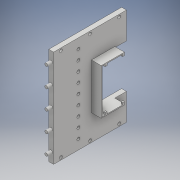
# Autodesk Inventor part: Front Plate V3
Saved by Autodesk Inventor 2017.3 (Build 213256000, 256)
## iProperties
Created: 2018-03-06
Part Number: Front Plate V3
Material: Generic
Document SubType Name: Modeling
Designer: Harsh Gupta
Density: 1 g/cm^3
Appearance: Default
Author: Harsh Gupta
Autodesk Inventor part; units mm, degrees
ref_plane "YZ Plane" through (0, 0, 0) normal (1, 0, 0) x (0, 1, 0)
sketch "Sketch2" plane through (0, 0, 0) normal (0, 1, 0) x (-1, 0, 0)
  line L0 (0, 0) -> (5, 0)
  line L1 (5, 0) -> (5, -100)
  line L2 (5, -100) -> (0, -100)
  line L3 (0, -100) -> (0, 0)
  dimension "d0" = 5
  dimension "d1" = 100
  constraints: 8 end point, 2 parallel, 1 horizontal, 1 perpendicular
  measures "d0" distance of L1.end L2.end
  measures "d1" distance of L0.end L1.end
extrude "Extrusion1" add sketch "Sketch2" along normal blind 75
sketch "Sketch4" plane through (0, 0, 0) normal (1, 0, 0) x (0, 0, -1)
  line L0 (0, 75) -> (100, 75) projected
  line L1 (27.5, 40) -> (72.5, 40)
  line L2 (72.5, 40) -> (72.5, 75)
  line L3 (72.5, 75) -> (27.5, 75)
  line L4 (27.5, 75) -> (27.5, 40)
  line L5 (100, 0) -> (100, 75) projected
  line L6 (0, 0) -> (100, 0) projected
  line L7 (0, 0) -> (0, 75) projected
  dimension "d9" = 27.5
  dimension "d11" = 40
  dimension "d12" = 45
  dimension "d13" = 27.5
  constraints: 8 end point, 2 parallel, 1 horizontal, 1 perpendicular, 1 point on line
  measures "d9" distance between parallel lines of L5 L2
  measures "d11" distance between parallel lines of L6 L1
  measures "d12" distance of L1.start L1.end
  measures "d13" distance between parallel lines of L7 L4
extrude "Extrusion3" cut sketch "Sketch4" against normal through all contours L0 L2 L1 L4
sketch "Sketch5" plane through (0, 0, 0) normal (1, 0, 0) x (0, 0, -1)
  line L0 (72.5, 43) -> (27.5, 43) projected
  line L1 (72.5, 63) -> (72.5, 43) projected
  line L2 (27.5, 63) -> (72.5, 63) projected
  line L3 (27.5, 43) -> (27.5, 63) projected
  circle A0 centre (28.5, 44) radius 0.75 projected
  circle A1 centre (28.5, 62) radius 0.75 projected
  circle A2 centre (71.5, 44) radius 0.75 projected
  circle A3 centre (71.5, 62) radius 0.75 projected
  line L4 (47.55, 45.5) -> (47.35, 45.5) projected
  line L5 (47.55, 45.5) -> (47.65, 45.6) projected
  line L6 (49.8, 45.6) -> (47.65, 45.6) projected
  line L7 (49.8, 45.6) -> (49.9, 45.5) projected
  line L8 (50.1, 45.5) -> (49.9, 45.5) projected
  line L9 (50.1, 45.5) -> (50.2, 45.6) projected
  line L10 (52.35, 45.6) -> (50.2, 45.6) projected
  line L11 (52.35, 45.6) -> (52.45, 45.5) projected
  line L12 (52.65, 45.5) -> (52.45, 45.5) projected
  line L13 (52.65, 45.5) -> (52.75, 45.6) projected
  line L14 (54.9, 45.6) -> (52.75, 45.6) projected
  line L15 (54.9, 45.6) -> (55, 45.5) projected
  line L16 (55, 43.2) -> (55, 45.5) projected
  line L17 (55, 43.2) -> (54.9, 43.1) projected
  line L18 (52.75, 43.1) -> (54.9, 43.1) projected
  line L19 (52.75, 43.1) -> (52.65, 43.2) projected
  line L20 (52.45, 43.2) -> (52.65, 43.2) projected
  line L21 (52.45, 43.2) -> (52.35, 43.1) projected
  line L22 (50.2, 43.1) -> (52.35, 43.1) projected
  line L23 (50.2, 43.1) -> (50.1, 43.2) projected
  line L24 (49.9, 43.2) -> (50.1, 43.2) projected
  line L25 (49.9, 43.2) -> (49.8, 43.1) projected
  line L26 (47.65, 43.1) -> (49.8, 43.1) projected
  line L27 (47.65, 43.1) -> (47.55, 43.2) projected
  line L28 (47.35, 43.2) -> (47.55, 43.2) projected
  line L29 (47.35, 43.2) -> (47.25, 43.1) projected
  line L30 (45.1, 43.1) -> (47.25, 43.1) projected
  line L31 (45.1, 43.1) -> (45, 43.2) projected
  line L32 (45, 45.5) -> (45, 43.2) projected
  line L33 (45, 45.5) -> (45.1, 45.6) projected
  line L34 (47.25, 45.6) -> (45.1, 45.6) projected
  line L35 (47.25, 45.6) -> (47.35, 45.5) projected
  line L36 (29, 56.95) -> (29, 56.75) projected
  line L37 (29.1, 56.95) -> (29, 56.95) projected
  line L38 (29.1, 56.75) -> (29.1, 56.95) projected
  line L39 (29, 56.75) -> (29.1, 56.75) projected
  line L40 (33.9, 56.95) -> (33.9, 56.75) projected
  line L41 (34, 56.95) -> (33.9, 56.95) projected
  line L42 (34, 56.75) -> (34, 56.95) projected
  line L43 (33.9, 56.75) -> (34, 56.75) projected
  line L44 (29, 55.8071) -> (29, 55.6071) projected
  line L45 (29.1, 55.8071) -> (29, 55.8071) projected
  line L46 (29.1, 55.6071) -> (29.1, 55.8071) projected
  line L47 (29, 55.6071) -> (29.1, 55.6071) projected
  line L48 (33.9, 55.8071) -> (33.9, 55.6071) projected
  line L49 (34, 55.8071) -> (33.9, 55.8071) projected
  line L50 (34, 55.6071) -> (34, 55.8071) projected
  line L51 (33.9, 55.6071) -> (34, 55.6071) projected
  line L52 (29, 54.6643) -> (29, 54.4643) projected
  line L53 (29.1, 54.6643) -> (29, 54.6643) projected
  line L54 (29.1, 54.4643) -> (29.1, 54.6643) projected
  line L55 (29, 54.4643) -> (29.1, 54.4643) projected
  line L56 (33.9, 54.6643) -> (33.9, 54.4643) projected
  line L57 (34, 54.6643) -> (33.9, 54.6643) projected
  line L58 (34, 54.4643) -> (34, 54.6643) projected
  line L59 (33.9, 54.4643) -> (34, 54.4643) projected
  line L60 (29, 53.5214) -> (29, 53.3214) projected
  line L61 (29.1, 53.5214) -> (29, 53.5214) projected
  line L62 (29.1, 53.3214) -> (29.1, 53.5214) projected
  line L63 (29, 53.3214) -> (29.1, 53.3214) projected
  line L64 (33.9, 53.5214) -> (33.9, 53.3214) projected
  line L65 (34, 53.5214) -> (33.9, 53.5214) projected
  line L66 (34, 53.3214) -> (34, 53.5214) projected
  line L67 (33.9, 53.3214) -> (34, 53.3214) projected
  line L68 (29, 52.3786) -> (29, 52.1786) projected
  line L69 (29.1, 52.3786) -> (29, 52.3786) projected
  line L70 (29.1, 52.1786) -> (29.1, 52.3786) projected
  line L71 (29, 52.1786) -> (29.1, 52.1786) projected
  line L72 (33.9, 52.3786) -> (33.9, 52.1786) projected
  line L73 (34, 52.3786) -> (33.9, 52.3786) projected
  line L74 (34, 52.1786) -> (34, 52.3786) projected
  line L75 (33.9, 52.1786) -> (34, 52.1786) projected
  line L76 (29, 51.2357) -> (29, 51.0357) projected
  line L77 (29.1, 51.2357) -> (29, 51.2357) projected
  line L78 (29.1, 51.0357) -> (29.1, 51.2357) projected
  line L79 (29, 51.0357) -> (29.1, 51.0357) projected
  line L80 (33.9, 51.2357) -> (33.9, 51.0357) projected
  line L81 (34, 51.2357) -> (33.9, 51.2357) projected
  line L82 (34, 51.0357) -> (34, 51.2357) projected
  line L83 (33.9, 51.0357) -> (34, 51.0357) projected
  line L84 (29, 50.0929) -> (29, 49.8929) projected
  line L85 (29.1, 50.0929) -> (29, 50.0929) projected
  line L86 (29.1, 49.8929) -> (29.1, 50.0929) projected
  line L87 (29, 49.8929) -> (29.1, 49.8929) projected
  line L88 (33.9, 50.0929) -> (33.9, 49.8929) projected
  line L89 (34, 50.0929) -> (33.9, 50.0929) projected
  line L90 (34, 49.8929) -> (34, 50.0929) projected
  line L91 (33.9, 49.8929) -> (34, 49.8929) projected
  line L92 (29, 48.95) -> (29, 48.75) projected
  line L93 (29.1, 48.95) -> (29, 48.95) projected
  line L94 (29.1, 48.75) -> (29.1, 48.95) projected
  line L95 (29, 48.75) -> (29.1, 48.75) projected
  line L96 (33.9, 48.95) -> (33.9, 48.75) projected
  line L97 (34, 48.95) -> (33.9, 48.95) projected
  line L98 (34, 48.75) -> (34, 48.95) projected
  line L99 (33.9, 48.75) -> (34, 48.75) projected
  line L100 (45.95, 50.5) -> (46.15, 50.5) projected
  line L101 (45.95, 50.55) -> (45.95, 50.5) projected
  line L102 (46.15, 50.55) -> (45.95, 50.55) projected
  line L103 (46.15, 50.5) -> (46.15, 50.55) projected
  line L104 (46.15, 55.5) -> (45.95, 55.5) projected
  line L105 (46.15, 55.45) -> (46.15, 55.5) projected
  line L106 (45.95, 55.45) -> (46.15, 55.45) projected
  line L107 (45.95, 55.5) -> (45.95, 55.45) projected
  line L108 (47.2667, 50.5) -> (47.4667, 50.5) projected
  line L109 (47.2667, 50.55) -> (47.2667, 50.5) projected
  line L110 (47.4667, 50.55) -> (47.2667, 50.55) projected
  line L111 (47.4667, 50.5) -> (47.4667, 50.55) projected
  line L112 (47.4667, 55.5) -> (47.2667, 55.5) projected
  line L113 (47.4667, 55.45) -> (47.4667, 55.5) projected
  line L114 (47.2667, 55.45) -> (47.4667, 55.45) projected
  line L115 (47.2667, 55.5) -> (47.2667, 55.45) projected
  line L116 (48.5833, 50.5) -> (48.7833, 50.5) projected
  line L117 (48.5833, 50.55) -> (48.5833, 50.5) projected
  line L118 (48.7833, 50.55) -> (48.5833, 50.55) projected
  line L119 (48.7833, 50.5) -> (48.7833, 50.55) projected
  line L120 (48.7833, 55.5) -> (48.5833, 55.5) projected
  line L121 (48.7833, 55.45) -> (48.7833, 55.5) projected
  line L122 (48.5833, 55.45) -> (48.7833, 55.45) projected
  line L123 (48.5833, 55.5) -> (48.5833, 55.45) projected
  line L124 (49.9, 50.5) -> (50.1, 50.5) projected
  line L125 (49.9, 50.55) -> (49.9, 50.5) projected
  line L126 (50.1, 50.55) -> (49.9, 50.55) projected
  line L127 (50.1, 50.5) -> (50.1, 50.55) projected
  line L128 (50.1, 55.5) -> (49.9, 55.5) projected
  line L129 (50.1, 55.45) -> (50.1, 55.5) projected
  line L130 (49.9, 55.45) -> (50.1, 55.45) projected
  line L131 (49.9, 55.5) -> (49.9, 55.45) projected
  line L132 (51.2167, 50.5) -> (51.4167, 50.5) projected
  line L133 (51.2167, 50.55) -> (51.2167, 50.5) projected
  line L134 (51.4167, 50.55) -> (51.2167, 50.55) projected
  line L135 (51.4167, 50.5) -> (51.4167, 50.55) projected
  line L136 (51.4167, 55.5) -> (51.2167, 55.5) projected
  line L137 (51.4167, 55.45) -> (51.4167, 55.5) projected
  line L138 (51.2167, 55.45) -> (51.4167, 55.45) projected
  line L139 (51.2167, 55.5) -> (51.2167, 55.45) projected
  line L140 (52.5333, 50.5) -> (52.7333, 50.5) projected
  line L141 (52.5333, 50.55) -> (52.5333, 50.5) projected
  line L142 (52.7333, 50.55) -> (52.5333, 50.55) projected
  line L143 (52.7333, 50.5) -> (52.7333, 50.55) projected
  line L144 (52.7333, 55.5) -> (52.5333, 55.5) projected
  line L145 (52.7333, 55.45) -> (52.7333, 55.5) projected
  line L146 (52.5333, 55.45) -> (52.7333, 55.45) projected
  line L147 (52.5333, 55.5) -> (52.5333, 55.45) projected
  line L148 (53.85, 50.5) -> (54.05, 50.5) projected
  line L149 (53.85, 50.55) -> (53.85, 50.5) projected
  line L150 (54.05, 50.55) -> (53.85, 50.55) projected
  line L151 (54.05, 50.5) -> (54.05, 50.55) projected
  line L152 (54.05, 55.5) -> (53.85, 55.5) projected
  line L153 (54.05, 55.45) -> (54.05, 55.5) projected
  line L154 (53.85, 55.45) -> (54.05, 55.45) projected
  line L155 (53.85, 55.5) -> (53.85, 55.45) projected
  line L156 (64.1, 50.5) -> (64.3, 50.5) projected
  line L157 (64.1, 50.55) -> (64.1, 50.5) projected
  line L158 (64.3, 50.55) -> (64.1, 50.55) projected
  line L159 (64.3, 50.5) -> (64.3, 50.55) projected
  line L160 (64.3, 55.5) -> (64.1, 55.5) projected
  line L161 (64.3, 55.45) -> (64.3, 55.5) projected
  line L162 (64.1, 55.45) -> (64.3, 55.45) projected
  line L163 (64.1, 55.5) -> (64.1, 55.45) projected
  line L164 (65.4167, 50.5) -> (65.6167, 50.5) projected
  line L165 (65.4167, 50.55) -> (65.4167, 50.5) projected
  line L166 (65.6167, 50.55) -> (65.4167, 50.55) projected
  line L167 (65.6167, 50.5) -> (65.6167, 50.55) projected
  line L168 (65.6167, 55.5) -> (65.4167, 55.5) projected
  line L169 (65.6167, 55.45) -> (65.6167, 55.5) projected
  line L170 (65.4167, 55.45) -> (65.6167, 55.45) projected
  line L171 (65.4167, 55.5) -> (65.4167, 55.45) projected
  line L172 (66.7333, 50.5) -> (66.9333, 50.5) projected
  line L173 (66.7333, 50.55) -> (66.7333, 50.5) projected
  line L174 (66.9333, 50.55) -> (66.7333, 50.55) projected
  line L175 (66.9333, 50.5) -> (66.9333, 50.55) projected
  line L176 (66.9333, 55.5) -> (66.7333, 55.5) projected
  line L177 (66.9333, 55.45) -> (66.9333, 55.5) projected
  line L178 (66.7333, 55.45) -> (66.9333, 55.45) projected
  line L179 (66.7333, 55.5) -> (66.7333, 55.45) projected
  line L180 (68.05, 50.5) -> (68.25, 50.5) projected
  line L181 (68.05, 50.55) -> (68.05, 50.5) projected
  line L182 (68.25, 50.55) -> (68.05, 50.55) projected
  line L183 (68.25, 50.5) -> (68.25, 50.55) projected
  line L184 (68.25, 55.5) -> (68.05, 55.5) projected
  line L185 (68.25, 55.45) -> (68.25, 55.5) projected
  line L186 (68.05, 55.45) -> (68.25, 55.45) projected
  line L187 (68.05, 55.5) -> (68.05, 55.45) projected
  line L188 (69.3667, 50.5) -> (69.5667, 50.5) projected
  line L189 (69.3667, 50.55) -> (69.3667, 50.5) projected
  line L190 (69.5667, 50.55) -> (69.3667, 50.55) projected
  line L191 (69.5667, 50.5) -> (69.5667, 50.55) projected
  line L192 (69.5667, 55.5) -> (69.3667, 55.5) projected
  line L193 (69.5667, 55.45) -> (69.5667, 55.5) projected
  line L194 (69.3667, 55.45) -> (69.5667, 55.45) projected
  line L195 (69.3667, 55.5) -> (69.3667, 55.45) projected
  line L196 (70.6833, 50.5) -> (70.8833, 50.5) projected
  line L197 (70.6833, 50.55) -> (70.6833, 50.5) projected
  line L198 (70.8833, 50.55) -> (70.6833, 50.55) projected
  line L199 (70.8833, 50.5) -> (70.8833, 50.55) projected
  line L200 (70.8833, 55.5) -> (70.6833, 55.5) projected
  line L201 (70.8833, 55.45) -> (70.8833, 55.5) projected
  line L202 (70.6833, 55.45) -> (70.8833, 55.45) projected
  line L203 (70.6833, 55.5) -> (70.6833, 55.45) projected
  line L204 (72, 50.5) -> (72.2, 50.5) projected
  line L205 (72, 50.55) -> (72, 50.5) projected
  line L206 (72.2, 50.55) -> (72, 50.55) projected
  line L207 (72.2, 50.5) -> (72.2, 50.55) projected
  line L208 (72.2, 55.5) -> (72, 55.5) projected
  line L209 (72.2, 55.45) -> (72.2, 55.5) projected
  line L210 (72, 55.45) -> (72.2, 55.45) projected
  line L211 (72, 55.5) -> (72, 55.45) projected
  line L212 (63.9, 55) -> (63.9, 51) projected
  line L213 (72.4, 55) -> (63.9, 55) projected
  line L214 (72.4, 51) -> (72.4, 55) projected
  line L215 (63.9, 51) -> (72.4, 51) projected
  line L216 (54.25, 51) -> (54.25, 55) projected
  line L217 (45.75, 51) -> (54.25, 51) projected
  line L218 (45.75, 55) -> (45.75, 51) projected
  line L219 (54.25, 55) -> (45.75, 55) projected
  line L220 (29.5, 57.75) -> (29.5, 48.25) projected
  line L221 (33.5, 57.75) -> (29.5, 57.75) projected
  line L222 (33.5, 48.25) -> (33.5, 57.75) projected
  line L223 (29.5, 48.25) -> (33.5, 48.25) projected
  line L224 (27.5, 63) -> (26.5, 63)
  line L225 (27.5, 40) -> (27.5, 75) projected
  line L226 (27.5, 63) -> (28.5, 63) construction
  line L227 (26.5, 63) -> (26.5, 39)
  line L228 (26.5, 39) -> (73.5, 39)
  line L229 (73.5, 39) -> (73.5, 63)
  line L230 (73.5, 63) -> (72.5, 63)
  line L231 (72.5, 75) -> (72.5, 40) projected
  line L232 (72.5, 40) -> (27.5, 40)
  line L233 (27.5, 40) -> (27.5, 63)
  point P0 (0, 0)
  dimension "d16" = 1
  dimension "d17" = 180
  dimension "d18" = 24
  dimension "d19" = 90
  dimension "d20" = 47
  dimension "d21" = 90
  constraints: 16 end point, 4 perpendicular, 2 horizontal, 2 parallel, 1 collinear, 1 point on line
  measures "d16" distance of L2.start L224.end
  measures "d17" angle of L224 L226
  measures "d18" distance of L224.end L227.end
  measures "d19" angle of L227 L224
  measures "d20" distance of L227.end L228.end
  measures "d21" angle of L228 L227
extrude "Extrusion4" add sketch "Sketch5" along normal blind 10 contours L1 L230 L229 L228 L227 L224 L3 L225 L232 L231
ref_plane "Work Plane1" through (8.5, -17.3753, -50) normal (1, 0, 0) x (0, 0, -1)
sketch "Sketch6" plane through (8.5, -17.3753, -50) normal (1, 0, 0) x (0, 0, -1)
  line L0 (22.5, 60.3753) -> (-22.5, 60.3753) projected
  line L1 (22.5, 80.3753) -> (22.5, 60.3753) projected
  line L2 (-22.5, 80.3753) -> (22.5, 80.3753) projected
  line L3 (-22.5, 60.3753) -> (-22.5, 80.3753) projected
  circle A0 centre (-21.5, 61.3753) radius 0.75 projected
  circle A1 centre (-21.5, 79.3753) radius 0.75 projected
  circle A2 centre (21.5, 61.3753) radius 0.75 projected
  circle A3 centre (21.5, 79.3753) radius 0.75 projected
  line L4 (-2.45, 62.8753) -> (-2.65, 62.8753) projected
  line L5 (-2.45, 62.8753) -> (-2.35, 62.9753) projected
  line L6 (-0.2, 62.9753) -> (-2.35, 62.9753) projected
  line L7 (-0.2, 62.9753) -> (-0.1, 62.8753) projected
  line L8 (0.1, 62.8753) -> (-0.1, 62.8753) projected
  line L9 (0.1, 62.8753) -> (0.2, 62.9753) projected
  line L10 (2.35, 62.9753) -> (0.2, 62.9753) projected
  line L11 (2.35, 62.9753) -> (2.45, 62.8753) projected
  line L12 (2.65, 62.8753) -> (2.45, 62.8753) projected
  line L13 (2.65, 62.8753) -> (2.75, 62.9753) projected
  line L14 (4.9, 62.9753) -> (2.75, 62.9753) projected
  line L15 (4.9, 62.9753) -> (5, 62.8753) projected
  line L16 (5, 60.5753) -> (5, 62.8753) projected
  line L17 (5, 60.5753) -> (4.9, 60.4753) projected
  line L18 (2.75, 60.4753) -> (4.9, 60.4753) projected
  line L19 (2.75, 60.4753) -> (2.65, 60.5753) projected
  line L20 (2.45, 60.5753) -> (2.65, 60.5753) projected
  line L21 (2.45, 60.5753) -> (2.35, 60.4753) projected
  line L22 (0.2, 60.4753) -> (2.35, 60.4753) projected
  line L23 (0.2, 60.4753) -> (0.1, 60.5753) projected
  line L24 (-0.1, 60.5753) -> (0.1, 60.5753) projected
  line L25 (-0.1, 60.5753) -> (-0.2, 60.4753) projected
  line L26 (-2.35, 60.4753) -> (-0.2, 60.4753) projected
  line L27 (-2.35, 60.4753) -> (-2.45, 60.5753) projected
  line L28 (-2.65, 60.5753) -> (-2.45, 60.5753) projected
  line L29 (-2.65, 60.5753) -> (-2.75, 60.4753) projected
  line L30 (-4.9, 60.4753) -> (-2.75, 60.4753) projected
  line L31 (-4.9, 60.4753) -> (-5, 60.5753) projected
  line L32 (-5, 62.8753) -> (-5, 60.5753) projected
  line L33 (-5, 62.8753) -> (-4.9, 62.9753) projected
  line L34 (-2.75, 62.9753) -> (-4.9, 62.9753) projected
  line L35 (-2.75, 62.9753) -> (-2.65, 62.8753) projected
  line L36 (-21, 74.3253) -> (-21, 74.1253) projected
  line L37 (-20.9, 74.3253) -> (-21, 74.3253) projected
  line L38 (-20.9, 74.1253) -> (-20.9, 74.3253) projected
  line L39 (-21, 74.1253) -> (-20.9, 74.1253) projected
  line L40 (-16.1, 74.3253) -> (-16.1, 74.1253) projected
  line L41 (-16, 74.3253) -> (-16.1, 74.3253) projected
  line L42 (-16, 74.1253) -> (-16, 74.3253) projected
  line L43 (-16.1, 74.1253) -> (-16, 74.1253) projected
  line L44 (-21, 73.1824) -> (-21, 72.9824) projected
  line L45 (-20.9, 73.1824) -> (-21, 73.1824) projected
  line L46 (-20.9, 72.9824) -> (-20.9, 73.1824) projected
  line L47 (-21, 72.9824) -> (-20.9, 72.9824) projected
  line L48 (-16.1, 73.1824) -> (-16.1, 72.9824) projected
  line L49 (-16, 73.1824) -> (-16.1, 73.1824) projected
  line L50 (-16, 72.9824) -> (-16, 73.1824) projected
  line L51 (-16.1, 72.9824) -> (-16, 72.9824) projected
  line L52 (-21, 72.0396) -> (-21, 71.8396) projected
  line L53 (-20.9, 72.0396) -> (-21, 72.0396) projected
  line L54 (-20.9, 71.8396) -> (-20.9, 72.0396) projected
  line L55 (-21, 71.8396) -> (-20.9, 71.8396) projected
  line L56 (-16.1, 72.0396) -> (-16.1, 71.8396) projected
  line L57 (-16, 72.0396) -> (-16.1, 72.0396) projected
  line L58 (-16, 71.8396) -> (-16, 72.0396) projected
  line L59 (-16.1, 71.8396) -> (-16, 71.8396) projected
  line L60 (-21, 70.8967) -> (-21, 70.6967) projected
  line L61 (-20.9, 70.8967) -> (-21, 70.8967) projected
  line L62 (-20.9, 70.6967) -> (-20.9, 70.8967) projected
  line L63 (-21, 70.6967) -> (-20.9, 70.6967) projected
  line L64 (-16.1, 70.8967) -> (-16.1, 70.6967) projected
  line L65 (-16, 70.8967) -> (-16.1, 70.8967) projected
  line L66 (-16, 70.6967) -> (-16, 70.8967) projected
  line L67 (-16.1, 70.6967) -> (-16, 70.6967) projected
  line L68 (-21, 69.7538) -> (-21, 69.5538) projected
  line L69 (-20.9, 69.7538) -> (-21, 69.7538) projected
  line L70 (-20.9, 69.5538) -> (-20.9, 69.7538) projected
  line L71 (-21, 69.5538) -> (-20.9, 69.5538) projected
  line L72 (-16.1, 69.7538) -> (-16.1, 69.5538) projected
  line L73 (-16, 69.7538) -> (-16.1, 69.7538) projected
  line L74 (-16, 69.5538) -> (-16, 69.7538) projected
  line L75 (-16.1, 69.5538) -> (-16, 69.5538) projected
  line L76 (-21, 68.611) -> (-21, 68.411) projected
  line L77 (-20.9, 68.611) -> (-21, 68.611) projected
  line L78 (-20.9, 68.411) -> (-20.9, 68.611) projected
  line L79 (-21, 68.411) -> (-20.9, 68.411) projected
  line L80 (-16.1, 68.611) -> (-16.1, 68.411) projected
  line L81 (-16, 68.611) -> (-16.1, 68.611) projected
  line L82 (-16, 68.411) -> (-16, 68.611) projected
  line L83 (-16.1, 68.411) -> (-16, 68.411) projected
  line L84 (-21, 67.4681) -> (-21, 67.2681) projected
  line L85 (-20.9, 67.4681) -> (-21, 67.4681) projected
  line L86 (-20.9, 67.2681) -> (-20.9, 67.4681) projected
  line L87 (-21, 67.2681) -> (-20.9, 67.2681) projected
  line L88 (-16.1, 67.4681) -> (-16.1, 67.2681) projected
  line L89 (-16, 67.4681) -> (-16.1, 67.4681) projected
  line L90 (-16, 67.2681) -> (-16, 67.4681) projected
  line L91 (-16.1, 67.2681) -> (-16, 67.2681) projected
  line L92 (-21, 66.3253) -> (-21, 66.1253) projected
  line L93 (-20.9, 66.3253) -> (-21, 66.3253) projected
  line L94 (-20.9, 66.1253) -> (-20.9, 66.3253) projected
  line L95 (-21, 66.1253) -> (-20.9, 66.1253) projected
  line L96 (-16.1, 66.3253) -> (-16.1, 66.1253) projected
  line L97 (-16, 66.3253) -> (-16.1, 66.3253) projected
  line L98 (-16, 66.1253) -> (-16, 66.3253) projected
  line L99 (-16.1, 66.1253) -> (-16, 66.1253) projected
  line L100 (-4.05, 67.8753) -> (-3.85, 67.8753) projected
  line L101 (-4.05, 67.9253) -> (-4.05, 67.8753) projected
  line L102 (-3.85, 67.9253) -> (-4.05, 67.9253) projected
  line L103 (-3.85, 67.8753) -> (-3.85, 67.9253) projected
  line L104 (-3.85, 72.8753) -> (-4.05, 72.8753) projected
  line L105 (-3.85, 72.8253) -> (-3.85, 72.8753) projected
  line L106 (-4.05, 72.8253) -> (-3.85, 72.8253) projected
  line L107 (-4.05, 72.8753) -> (-4.05, 72.8253) projected
  line L108 (-2.7333, 67.8753) -> (-2.5333, 67.8753) projected
  line L109 (-2.7333, 67.9253) -> (-2.7333, 67.8753) projected
  line L110 (-2.5333, 67.9253) -> (-2.7333, 67.9253) projected
  line L111 (-2.5333, 67.8753) -> (-2.5333, 67.9253) projected
  line L112 (-2.5333, 72.8753) -> (-2.7333, 72.8753) projected
  line L113 (-2.5333, 72.8253) -> (-2.5333, 72.8753) projected
  line L114 (-2.7333, 72.8253) -> (-2.5333, 72.8253) projected
  line L115 (-2.7333, 72.8753) -> (-2.7333, 72.8253) projected
  line L116 (-1.4167, 67.8753) -> (-1.2167, 67.8753) projected
  line L117 (-1.4167, 67.9253) -> (-1.4167, 67.8753) projected
  line L118 (-1.2167, 67.9253) -> (-1.4167, 67.9253) projected
  line L119 (-1.2167, 67.8753) -> (-1.2167, 67.9253) projected
  line L120 (-1.2167, 72.8753) -> (-1.4167, 72.8753) projected
  line L121 (-1.2167, 72.8253) -> (-1.2167, 72.8753) projected
  line L122 (-1.4167, 72.8253) -> (-1.2167, 72.8253) projected
  line L123 (-1.4167, 72.8753) -> (-1.4167, 72.8253) projected
  line L124 (-0.1, 67.8753) -> (0.1, 67.8753) projected
  line L125 (-0.1, 67.9253) -> (-0.1, 67.8753) projected
  line L126 (0.1, 67.9253) -> (-0.1, 67.9253) projected
  line L127 (0.1, 67.8753) -> (0.1, 67.9253) projected
  line L128 (0.1, 72.8753) -> (-0.1, 72.8753) projected
  line L129 (0.1, 72.8253) -> (0.1, 72.8753) projected
  line L130 (-0.1, 72.8253) -> (0.1, 72.8253) projected
  line L131 (-0.1, 72.8753) -> (-0.1, 72.8253) projected
  line L132 (1.2167, 67.8753) -> (1.4167, 67.8753) projected
  line L133 (1.2167, 67.9253) -> (1.2167, 67.8753) projected
  line L134 (1.4167, 67.9253) -> (1.2167, 67.9253) projected
  line L135 (1.4167, 67.8753) -> (1.4167, 67.9253) projected
  line L136 (1.4167, 72.8753) -> (1.2167, 72.8753) projected
  line L137 (1.4167, 72.8253) -> (1.4167, 72.8753) projected
  line L138 (1.2167, 72.8253) -> (1.4167, 72.8253) projected
  line L139 (1.2167, 72.8753) -> (1.2167, 72.8253) projected
  line L140 (2.5333, 67.8753) -> (2.7333, 67.8753) projected
  line L141 (2.5333, 67.9253) -> (2.5333, 67.8753) projected
  line L142 (2.7333, 67.9253) -> (2.5333, 67.9253) projected
  line L143 (2.7333, 67.8753) -> (2.7333, 67.9253) projected
  line L144 (2.7333, 72.8753) -> (2.5333, 72.8753) projected
  line L145 (2.7333, 72.8253) -> (2.7333, 72.8753) projected
  line L146 (2.5333, 72.8253) -> (2.7333, 72.8253) projected
  line L147 (2.5333, 72.8753) -> (2.5333, 72.8253) projected
  line L148 (3.85, 67.8753) -> (4.05, 67.8753) projected
  line L149 (3.85, 67.9253) -> (3.85, 67.8753) projected
  line L150 (4.05, 67.9253) -> (3.85, 67.9253) projected
  line L151 (4.05, 67.8753) -> (4.05, 67.9253) projected
  line L152 (4.05, 72.8753) -> (3.85, 72.8753) projected
  line L153 (4.05, 72.8253) -> (4.05, 72.8753) projected
  line L154 (3.85, 72.8253) -> (4.05, 72.8253) projected
  line L155 (3.85, 72.8753) -> (3.85, 72.8253) projected
  line L156 (14.1, 67.8753) -> (14.3, 67.8753) projected
  line L157 (14.1, 67.9253) -> (14.1, 67.8753) projected
  line L158 (14.3, 67.9253) -> (14.1, 67.9253) projected
  line L159 (14.3, 67.8753) -> (14.3, 67.9253) projected
  line L160 (14.3, 72.8753) -> (14.1, 72.8753) projected
  line L161 (14.3, 72.8253) -> (14.3, 72.8753) projected
  line L162 (14.1, 72.8253) -> (14.3, 72.8253) projected
  line L163 (14.1, 72.8753) -> (14.1, 72.8253) projected
  line L164 (15.4167, 67.8753) -> (15.6167, 67.8753) projected
  line L165 (15.4167, 67.9253) -> (15.4167, 67.8753) projected
  line L166 (15.6167, 67.9253) -> (15.4167, 67.9253) projected
  line L167 (15.6167, 67.8753) -> (15.6167, 67.9253) projected
  line L168 (15.6167, 72.8753) -> (15.4167, 72.8753) projected
  line L169 (15.6167, 72.8253) -> (15.6167, 72.8753) projected
  line L170 (15.4167, 72.8253) -> (15.6167, 72.8253) projected
  line L171 (15.4167, 72.8753) -> (15.4167, 72.8253) projected
  line L172 (16.7333, 67.8753) -> (16.9333, 67.8753) projected
  line L173 (16.7333, 67.9253) -> (16.7333, 67.8753) projected
  line L174 (16.9333, 67.9253) -> (16.7333, 67.9253) projected
  line L175 (16.9333, 67.8753) -> (16.9333, 67.9253) projected
  line L176 (16.9333, 72.8753) -> (16.7333, 72.8753) projected
  line L177 (16.9333, 72.8253) -> (16.9333, 72.8753) projected
  line L178 (16.7333, 72.8253) -> (16.9333, 72.8253) projected
  line L179 (16.7333, 72.8753) -> (16.7333, 72.8253) projected
  line L180 (18.05, 67.8753) -> (18.25, 67.8753) projected
  line L181 (18.05, 67.9253) -> (18.05, 67.8753) projected
  line L182 (18.25, 67.9253) -> (18.05, 67.9253) projected
  line L183 (18.25, 67.8753) -> (18.25, 67.9253) projected
  line L184 (18.25, 72.8753) -> (18.05, 72.8753) projected
  line L185 (18.25, 72.8253) -> (18.25, 72.8753) projected
  line L186 (18.05, 72.8253) -> (18.25, 72.8253) projected
  line L187 (18.05, 72.8753) -> (18.05, 72.8253) projected
  line L188 (19.3667, 67.8753) -> (19.5667, 67.8753) projected
  line L189 (19.3667, 67.9253) -> (19.3667, 67.8753) projected
  line L190 (19.5667, 67.9253) -> (19.3667, 67.9253) projected
  line L191 (19.5667, 67.8753) -> (19.5667, 67.9253) projected
  line L192 (19.5667, 72.8753) -> (19.3667, 72.8753) projected
  line L193 (19.5667, 72.8253) -> (19.5667, 72.8753) projected
  line L194 (19.3667, 72.8253) -> (19.5667, 72.8253) projected
  line L195 (19.3667, 72.8753) -> (19.3667, 72.8253) projected
  line L196 (20.6833, 67.8753) -> (20.8833, 67.8753) projected
  line L197 (20.6833, 67.9253) -> (20.6833, 67.8753) projected
  line L198 (20.8833, 67.9253) -> (20.6833, 67.9253) projected
  line L199 (20.8833, 67.8753) -> (20.8833, 67.9253) projected
  line L200 (20.8833, 72.8753) -> (20.6833, 72.8753) projected
  line L201 (20.8833, 72.8253) -> (20.8833, 72.8753) projected
  line L202 (20.6833, 72.8253) -> (20.8833, 72.8253) projected
  line L203 (20.6833, 72.8753) -> (20.6833, 72.8253) projected
  line L204 (22, 67.8753) -> (22.2, 67.8753) projected
  line L205 (22, 67.9253) -> (22, 67.8753) projected
  line L206 (22.2, 67.9253) -> (22, 67.9253) projected
  line L207 (22.2, 67.8753) -> (22.2, 67.9253) projected
  line L208 (22.2, 72.8753) -> (22, 72.8753) projected
  line L209 (22.2, 72.8253) -> (22.2, 72.8753) projected
  line L210 (22, 72.8253) -> (22.2, 72.8253) projected
  line L211 (22, 72.8753) -> (22, 72.8253) projected
  line L212 (13.9, 72.3753) -> (13.9, 68.3753) projected
  line L213 (22.4, 72.3753) -> (13.9, 72.3753) projected
  line L214 (22.4, 68.3753) -> (22.4, 72.3753) projected
  line L215 (13.9, 68.3753) -> (22.4, 68.3753) projected
  line L216 (4.25, 68.3753) -> (4.25, 72.3753) projected
  line L217 (-4.25, 68.3753) -> (4.25, 68.3753) projected
  line L218 (-4.25, 72.3753) -> (-4.25, 68.3753) projected
  line L219 (4.25, 72.3753) -> (-4.25, 72.3753) projected
  line L220 (-20.5, 75.1253) -> (-20.5, 65.6253) projected
  line L221 (-16.5, 75.1253) -> (-20.5, 75.1253) projected
  line L222 (-16.5, 65.6253) -> (-16.5, 75.1253) projected
  line L223 (-20.5, 65.6253) -> (-16.5, 65.6253) projected
  line L224 (-22.5, 80.3753) -> (-20.5, 80.3753)
  line L225 (-20.5, 80.3753) -> (-20.5, 78.3753)
  line L226 (-20.5, 78.3753) -> (-22.5, 78.3753)
  line L227 (-22.5, 78.3753) -> (-22.5, 80.3753)
  line L228 (-22.5, 60.3753) -> (-20.5, 60.3753)
  line L229 (-20.5, 60.3753) -> (-20.5, 62.3753)
  line L230 (-20.5, 62.3753) -> (-22.5, 62.3753)
  line L231 (-22.5, 62.3753) -> (-22.5, 60.3753)
  line L232 (22.5, 60.3753) -> (20.5, 60.3753)
  line L233 (20.5, 60.3753) -> (20.5, 62.3753)
  line L234 (20.5, 62.3753) -> (22.5, 62.3753)
  line L235 (22.5, 62.3753) -> (22.5, 60.3753)
  line L236 (22.5, 80.3753) -> (20.5, 80.3753)
  line L237 (20.5, 80.3753) -> (20.5, 78.3753)
  line L238 (20.5, 78.3753) -> (22.5, 78.3753)
  line L239 (22.5, 78.3753) -> (22.5, 80.3753)
  point P0 (-50, 17.3753)
  dimension "d24" = 2
  dimension "d25" = 2
  dimension "d26" = 2
  dimension "d27" = 2
  dimension "d28" = 2
  dimension "d29" = 2
  dimension "d30" = 2
  dimension "d31" = 2
  constraints: 32 end point, 8 parallel, 4 horizontal, 4 perpendicular
  measures "d24" distance of L225.end L226.end
  measures "d25" distance of L224.end L225.end
  measures "d26" distance of L230.end L229.end
  measures "d27" distance of L229.end L228.end
  measures "d28" distance of L233.end L234.end
  measures "d29" distance of L232.end L233.end
  measures "d30" distance of L238.end L237.end
  measures "d31" distance of L237.end L236.end
extrude "Extrusion5" add sketch "Sketch6" along normal up to surface (1.5 mm away) contours L0 L233 L234 L1 | L0 L3 L230 L229 | L238 L237 L2 L1 | L3 L2 L225 L226 | A0 | A1 | A2 | A3
sketch "Sketch8" plane through (0, 0, 0) normal (0, -1, 0) x (1, 0, 0)
  circle A0 centre (-2.5, -10) radius 1.5
  line L0 (-5, 0) -> (-5, -100) projected
  line L1 (0, 0) -> (-5, 0) projected
  dimension "d36" = 3
  dimension "d37" = 2.5
  dimension "d38" = 10
  constraints: 1 centre point
  measures "d36" diameter of A0
  measures "d37" distance from line of L0 A0.centre
  measures "d38" distance from line of A0.centre L1
extrude "Extrusion7" add sketch "Sketch8" along normal blind 5
pattern_linear "Rectangular Pattern1" count 5 spacing 20 along (0, 0, -1) of "Extrusion7"
sketch "Sketch9" plane through (0, 0, 0) normal (1, 0, 0) x (0, 0, -1)
  line L0 (100, 0) -> (100, 75) projected
  line L1 (0, 23) -> (100, 23)
  line L2 (100, 23) -> (100, 28)
  line L3 (100, 28) -> (0, 28)
  line L4 (0, 28) -> (0, 23)
  line L5 (100, 0) -> (0, 0) projected
  circle A0 centre (10, 25.5) radius 1.5
  line L6 (0, 75) -> (27.5, 75) projected
  line L7 (0, 0) -> (5, 0)
  line L8 (5, 0) -> (5, 75)
  line L9 (5, 75) -> (0, 75)
  line L10 (0, 75) -> (0, 0)
  dimension "d44" = 5
  dimension "d45" = 23
  dimension "d46" = 3
  dimension "d47" = 2.5
  dimension "d54" = 5
  dimension "d55" = 5
  constraints: 16 end point, 4 parallel, 2 horizontal, 2 perpendicular, 2 point on line, 1 centre point
  measures "d44" distance of L2.end L1.end
  measures "d45" distance between parallel lines of L5 L1
  measures "d46" diameter of A0
  measures "d47" distance from line of L1 A0.centre
  measures "d54" distance of L9.end L8.end
  measures "d55" distance from line of L8 A0.centre
extrude "Extrusion8" cut sketch "Sketch9" against normal blind 2.5 contours A0
pattern_linear "Rectangular Pattern2" count 9 spacing 10 along (0, 0, -1) of "Extrusion8"
sketch "Sketch10" plane through (0, 0, 0) normal (1, 0, 0) x (0, 0, -1)
  circle A0 centre (2.5, 7.5) radius 1.5
  line L0 (0, 0) -> (0, 75) projected
  line L1 (100, 0) -> (0, 0) projected
  dimension "d56" = 3
  dimension "d57" = 2.5
  dimension "d58" = 7.5
  constraints: 1 centre point
  measures "d56" diameter of A0
  measures "d57" distance from line of L0 A0.centre
  measures "d58" distance from line of L1 A0.centre
extrude "Extrusion9" cut sketch "Sketch10" against normal blind 2.5
pattern_linear "Rectangular Pattern3" count 3 spacing 30 along (0, 1, 0) of "Extrusion9"
ref_plane "Work Plane2" through (-5, 0, -50) normal (0, 0, 1) x (1, 0, 0)
mirror "Mirror1" about plane through (-5, 0, -50) normal (0, 0, 1) of "Extrusion9", "Rectangular Pattern3"
sketch "Sketch7" plane through (-5, 0, -100) normal (-1, 0, 0) x (0, 0, 1)
  line L0 (30.2022, 30) -> (42.2022, 30) projected
  line L1 (42.2022, 30) -> (42.2022, 41) projected
  line L2 (30.2022, 41) -> (42.2022, 41) projected
  line L3 (30.2022, 30) -> (30.2022, 41) projected
  line L4 (33.2022, 40) -> (39.2022, 40) projected
  line L5 (39.2022, 40) -> (41.2022, 38) projected
  line L6 (41.2022, 38) -> (41.2022, 31) projected
  line L7 (41.2022, 31) -> (31.2022, 31) projected
  line L8 (31.2022, 31) -> (31.2022, 38) projected
  line L9 (31.2022, 38) -> (33.2022, 40) projected
  line L10 (68.7022, 30) -> (59.7022, 30) projected
  line L11 (68.7022, 30) -> (68.7022, 41) projected
  line L12 (59.7022, 41) -> (68.7022, 41) projected
  line L13 (59.7022, 30) -> (59.7022, 41) projected
  circle A0 centre (64.2022, 36.5) radius 3 projected
  line L14 (42.2022, 30) -> (30.2022, 30)
  line L15 (30.2022, 30) -> (30.2022, 40)
  line L16 (30.2022, 40) -> (42.2022, 40)
  line L17 (42.2022, 40) -> (42.2022, 30)
  line L18 (72.5, 40) -> (27.5, 40) projected
  line L19 (59.7022, 30) -> (68.7022, 30)
  line L20 (68.7022, 30) -> (68.7022, 40)
  line L21 (68.7022, 40) -> (59.7022, 40)
  line L22 (59.7022, 40) -> (59.7022, 30)
  point P0 (100, 0)
  constraints: 16 end point, 4 parallel, 3 point on line, 2 horizontal, 2 perpendicular, 1 collinear
equation "\"d9\" = d13"
body "Solid1"
